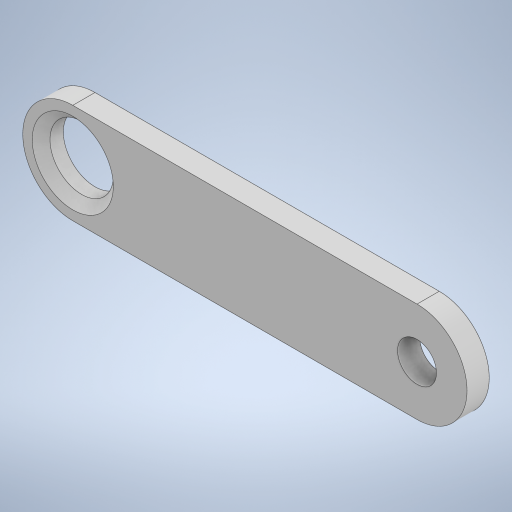
# Autodesk Inventor part: gripper_mechanism2
Saved by Autodesk Inventor 2023 (Build 270158000, 158)
## iProperties
Created: 2024-06-26
Part Number: gripper_mechanism2
Material: Generic
Document SubType Name: Modeling
Designer: Swoby
Density: 1 g/cm^3
Appearance: Default
Author: Swoby
Autodesk Inventor part; units mm, degrees
ref_plane "YZ Plane" through (0, 0, 0) normal (1, 0, 0) x (0, 1, 0)
ref_plane "XZ Plane" through (0, 0, 0) normal (0, 1, 0) x (-1, 0, 0)
ref_plane "XY Plane" through (0, 0, 0) normal (0, 0, 1) x (1, 0, 0)
sketch "Sketch1" plane through (0, 0, 0) normal (0, 0, 1) x (1, 0, 0)
  line L0 (-15.5, 0) -> (15.5, 0) construction
  line L1 (-15.5, -4.5) -> (15.5, -4.5)
  line L2 (15.5, 4.5) -> (-15.5, 4.5)
  arc A0 (-15.5, 4.5) -> (-15.5, -4.5) centre (-15.5, 0) ccw
  arc A1 (15.5, -4.5) -> (15.5, 4.5) centre (15.5, 0) ccw
  circle A2 centre (-15.5, 0) radius 2.85
  circle A3 centre (15.5, 0) radius 1.75
  point P0 (0, 0)
  point P1 (0, 0)
  dimension "d0" = 9
  dimension "d1" = 31
  dimension "d2" = 5.7
  dimension "d3" = 3.5
  constraints: 8 end point, 4 centre point, 4 point on circle, 4 tangent, 3 coincident, 1 horizontal, 1 midpoint, 1 parallel
  measures "d0" distance between parallel lines of L1 L2
  measures "d1" distance of L0.end L0.start
  measures "d2" diameter of A2
  measures "d3" diameter of A3
extrude "Extrusion1" add sketch "Sketch1" along normal blind 2
chamfer "Chamfer1" distance 0.8 angle 45 1 edges at (-18.35, 0, 2)
body "Solid1"
